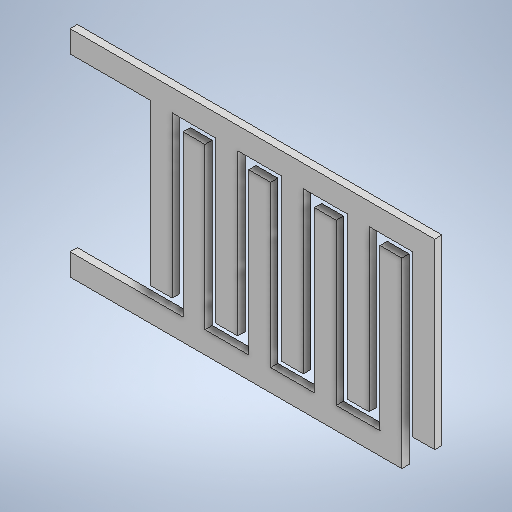
# Autodesk Inventor part: sensor_001_001
Saved by Autodesk Inventor 2025.2 (Build 292293000, 293)
## iProperties
Created: 2025-03-19
Part Number: sensor_001_001
Material: Genérico
Document SubType Name: Modeling
Designer: Carlos Dias
Density: 1 g/cm^3
Appearance: Padrão
Author: Carlos Dias
Autodesk Inventor part; units mm, degrees
ref_plane "YZ Plane" through (0, 0, 0) normal (1, 0, 0) x (0, 1, 0)
ref_plane "XZ Plane" through (0, 0, 0) normal (0, 1, 0) x (-1, 0, 0)
ref_plane "XY Plane" through (0, 0, 0) normal (0, 0, 1) x (1, 0, 0)
sketch "Esboço1" plane through (0, 0, 0) normal (0, 0, 1) x (1, 0, 0)
  line L0 (-25, 13) -> (-25, 10)
  line L1 (-25, 13) -> (25, 13)
  line L2 (25, 13) -> (25, -12)
  line L3 (25, -12) -> (22, -12)
  line L4 (22, -12) -> (22, 10)
  line L5 (22, 10) -> (16, 10)
  line L6 (-14, 10) -> (-25, 10)
  line L7 (-25, -13.5) -> (-9.5, -13.5)
  line L8 (-9.5, 8.5) -> (-9.5, -13.5)
  line L9 (-9.5, 8.5) -> (-6.5, 8.5)
  line L10 (-6.5, 8.5) -> (-6.5, -13.5)
  line L11 (-6.5, -13.5) -> (-0.5, -13.5)
  line L12 (-0.5, 8.5) -> (-0.5, -13.5)
  line L13 (-0.5, 8.5) -> (2.5, 8.5)
  line L14 (2.5, 8.5) -> (2.5, -13.5)
  line L15 (2.5, -13.5) -> (8.5, -13.5)
  line L16 (8.5, 8.5) -> (8.5, -13.5)
  line L17 (8.5, 8.5) -> (11.5, 8.5)
  line L18 (11.5, 8.5) -> (11.5, -13.5)
  line L19 (11.5, -13.5) -> (17.5, -13.5)
  line L20 (17.5, 8.5) -> (17.5, -13.5)
  line L21 (17.5, 8.5) -> (20.5, 8.5)
  line L22 (20.5, 8.5) -> (20.5, -13.5)
  line L23 (-25, -13.5) -> (-25, -16.5)
  line L24 (20.5, -13.5) -> (20.5, -16.5)
  line L25 (-25, -16.5) -> (20.5, -16.5)
  line L26 (16, 10) -> (16, -12)
  line L27 (13, -12) -> (16, -12)
  line L28 (13, 10) -> (13, -12)
  line L29 (7, 10) -> (13, 10)
  line L30 (7, 10) -> (7, -12)
  line L31 (4, -12) -> (7, -12)
  line L32 (4, 10) -> (4, -12)
  line L33 (-2, 10) -> (4, 10)
  line L34 (-2, 10) -> (-2, -12)
  line L35 (-5, -12) -> (-2, -12)
  line L36 (-5, 10) -> (-5, -12)
  line L37 (-11, 10) -> (-5, 10)
  line L38 (-11, 10) -> (-11, -12)
  line L39 (-14, -12) -> (-11, -12)
  line L40 (-14, 10) -> (-14, -12)
  point P0 (0, 0)
  point P1 (-25, 11.5)
  point P2 (0, 13)
  point P3 (23.5, -12)
  point P4 (-8, 8.5)
  point P5 (-3.5, -13.5)
  point P6 (-3.5, -12)
  dimension "d0" = 10
  dimension "d2" = 3
  dimension "d3" = 50
  dimension "d4" = 25
  dimension "d5" = 3
  dimension "d14" = 6
  dimension "d22" = 3
  dimension "d31" = 1.5
  dimension "d34" = 3
  dimension "d37" = 1.5
  dimension "d38" = 1.5
  dimension "d40" = 11
  constraints: 82 end point, 30 equal length, 21 vertical, 20 horizontal, 6 midpoint, 2 vertical alignment
  measures "d0" vertical distance of L0.end point (0, 0)
  measures "d2" distance of L0.start L0.end
  measures "d3" distance of L0.start L1.end
  measures "d4" distance of L1.end L2.end
  measures "d5" distance of L2.end L3.end
  measures "d14" distance of L4.end L5.end
  measures "d22" distance between parallel lines of L1 L5
  measures "d31" distance between parallel lines of L36 L10
  measures "d34" distance between parallel lines of L10 L8
  measures "d37" distance of point (-3.5, -13.5) point (-3.5, -12)
  measures "d38" distance between parallel lines of L5 L21
  measures "d40" distance of L6.start L0.end
extrude "Extrusão1" add sketch "Esboço1" along normal mid plane 1
